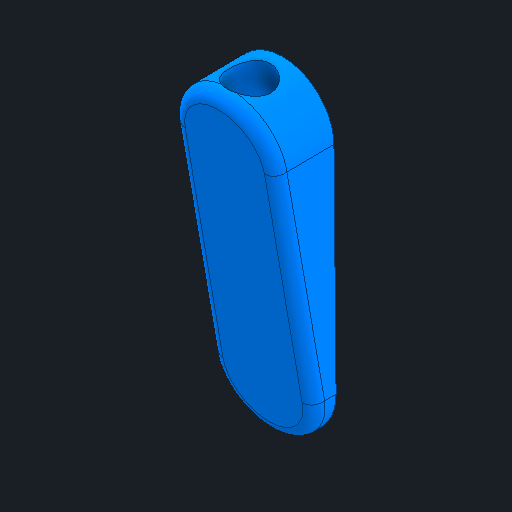
# Autodesk Inventor part: shaft_outlet
Saved by Autodesk Inventor 2023 (Build 270158030, 158C)
## iProperties
Created: 2022-03-28
Part Number: shaft_outlet
Material: Generic
Document SubType Name: Modeling
Designer: kardo
Density: 1 g/cm^3
Appearance: Blue Plastic
Author: kardo
Autodesk Inventor part; units mm, degrees
ref_plane "YZ Plane" through (0, 0, 0) normal (1, 0, 0) x (0, 1, 0)
ref_plane "XZ Plane" through (0, 0, 0) normal (0, 1, 0) x (-1, 0, 0)
ref_plane "XY Plane" through (0, 0, 0) normal (0, 0, 1) x (1, 0, 0)
derived "stencil_frame.ipt"
sketch "sk_drivetrain_profile" plane through (6, 0, 0) normal (1, 0, 0) x (0, 1, 0)
  line L0 (-529.1913, 0) -> (410.1479, 0) construction
  line L1 (-345, 3089.1136) -> (-345, -1866.0023) construction
  line L2 (0, 3089.1136) -> (0, -1866.0023) construction
  line L3 (-134.0777, 53.4546) -> (-127.3039, 26.2863)
  line L4 (-377, 0) -> (-313.1194, 3.9071)
  line L5 (-130.6908, 39.8704) -> (-224.6958, 16.4323)
  line L6 (-301.4275, 4.6222) -> (-262.5191, 7.002) construction
  line L7 (-262.5191, 7.002) -> (-224.6958, 16.4323) construction
  line L8 (-127.3039, 26.2863) -> (-127.3039, 21.2863) construction
  line L9 (-313.1194, 3.9071) -> (-301.4275, 4.6222)
  line L10 (-869.78, 3004.1953) -> (348.339, -1881.413) construction
  spline S0 degree 2 poles (-301.4275, 4.6222) (-262.5191, 7.002) (-224.6958, 16.4323) knots 1 1 1 2 2 2
  line L11 (-225.3679, 19.1279) -> (-131.3629, 42.566) construction
  line L12 (-130.0187, 37.1748) -> (-224.0238, 13.7367) construction
  line L13 (-225.3679, 19.1279) -> (-224.0238, 13.7367) construction
  line L14 (0, 21.3303) -> (-241.5001, 18.9703) construction
  line L15 (-49.1478, 22.05) -> (-303.2844, 19.5666) construction
  point P0 (0, 0)
  point P1 (-213.4159, 19.2447)
  point P2 (-201.4639, 19.3615)
  point P3 (-196.4544, 20.6106)
sketch "sk_prop_shaft_cut" plane through (6, 0, 21.3303) normal (0, -0.0097716, 0.9999523) x (0, -0.9999523, -0.0097716)
  line L0 (225.3787, -4.7781) -> (196.4521, -4.7781)
  line L1 (225.3787, 4.7781) -> (196.4521, 4.7781)
  arc A0 (196.4521, 4.7781) -> (196.4521, -4.7781) centre (196.4521, 0) ccw
  arc A1 (225.3787, -4.7781) -> (225.3787, 4.7781) centre (225.3787, 0) ccw
  point P0 (0.2084, -6)
  point P1 (213.4261, 0)
  point P2 (201.4736, 0)
ref_plane "plane_motor_mount" through (0, -120.75, 0) normal (0, 0.9702957, 0.2419219) x (-1, 0, 0)
derived "parameters_powertrain.ipt"
derived "parameters_frame.ipt"
extrude "lower_plate" add sketch "sk_prop_shaft_cut" along normal blind 1.2
sketch "sk_upper_plate" plane through (6, -225.3797, 20.3279) normal (0, -0.0097716, 0.9999523) x (1, 0, 0)
  line L0 (-4.7781, 28.9266) -> (-4.7781, 0) projected
  arc A0 (-4.7781, 0) -> (4.7781, 0) centre (0, 0) ccw projected
  line L1 (4.7781, 0) -> (4.7781, 28.9266) projected
  arc A1 (4.7781, 28.9266) -> (-4.7781, 28.9266) centre (0, 28.9266) ccw projected
  line L2 (-6.7781, 0) -> (-6.7781, 28.9266)
  arc A2 (6.7781, 28.9266) -> (-6.7781, 28.9266) centre (0, 28.9266) ccw
  line L3 (6.7781, 28.9266) -> (6.7781, 0)
  arc A3 (-6.7781, 0) -> (6.7781, 0) centre (0, 0) ccw
  point P0 (-6, 225.1703)
  dimension "d6" = 2
  constraints: 4 end point, 4 point on circle, 2 centre point, 3 other
  measures "d6" distance between parallel lines of L2 L0
extrude "upper_plate" add sketch "sk_upper_plate" along normal blind 8.89 contours A1 L1 A0 L0 | L2 A2 L3 A3
sketch "sk_trim" plane through (12.7781, -225.3797, 20.3279) normal (1, 0, 0) x (0, 0.0097716, -0.9999523)
  line L0 (-1.9447, -6.7781) -> (-8.89, 35.7047)
  line L1 (0, 0) -> (0, -6.7781) projected
  line L2 (-8.89, 35.7047) -> (-8.89, 28.9266) projected
  line L3 (0, -6.7781) -> (-1.9447, -6.7781)
  line L4 (-1.9447, -6.7781) -> (-8.89, -6.7781)
  line L5 (-8.89, -6.7781) -> (-8.89, 28.9266)
  dimension "d16" = 1.9447
  constraints: 8 end point, 2 collinear, 1 perpendicular
  measures "d16" distance of L1.end L0.start
extrude "trim" cut sketch "sk_trim" against normal through all
sketch "sk_drill" plane through (0, -120.75, 0) normal (0, 0.9702957, 0.2419219) x (-1, 0, 0)
  circle A0 centre (-6, 41.091) radius 2.7781
  point P0 (0, -29.2121)
  dimension "d9" = 5.5563
  constraints: 1 centre point, 1 coincident
  measures "d9" diameter of A0
extrude "drill" cut sketch "sk_drill" along normal through all both and the other way through all
fillet "Fillet1" radius 1.5 6 edges at (10.7929, -230.1945, 22.5502) (1.2071, -230.1945, 22.5502) (-0.7781, -210.97, 25.8863) (10.7929, -191.7455, 29.2224) (1.2071, -191.7455, 29.2224) (12.7781, -210.97, 25.8863)
equation "\"d4\" = shell_thickness"
equation "\"d7\" = 1.6 * prop_shaft_sleeve_od"
equation "\"d16\" = 0.35 * prop_shaft_sleeve_od"
equation "\"d9\" = prop_shaft_sleeve_od"
equation "\"shell_thickness\" = 1.2"
equation "\"prop_shaft_sleeve_od\" = 5.55625"
body "Solid1"
